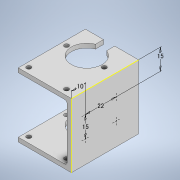
# Autodesk Inventor part: サーボモータ固定用２軸目3mm改_printer
Saved by Autodesk Inventor 2022 (Build 260153000, 153)
## iProperties
Created: 2022-11-23
Part Number: サーボモータ固定用２軸目3mm改_printer
Material: 一般
Document SubType Name: Modeling
Designer: tdn82
Density: 1 g/cm^3
Appearance: 既定
Author: tdn82
Autodesk Inventor part; units mm, degrees
ref_plane "YZ Plane" through (0, 0, 0) normal (1, 0, 0) x (0, 1, 0)
ref_plane "XZ Plane" through (0, 0, 0) normal (0, 1, 0) x (-1, 0, 0)
ref_plane "XY Plane" through (0, 0, 0) normal (0, 0, 1) x (1, 0, 0)
sketch "スケッチ1" plane through (0, 0, 0) normal (0, 1, 0) x (-1, 0, 0)
  line L0 (0, 0) -> (-38, 0)
  line L1 (-38, 0) -> (-38, -48)
  line L2 (-38, -48) -> (0, -48)
  line L3 (0, -48) -> (0, 0)
  dimension "d0" = 48
  dimension "d1" = 38
  constraints: 8 end point, 2 parallel, 1 horizontal, 1 perpendicular
  measures "d0" distance of L0.end L1.end
  measures "d1" distance of L1.end L2.end
extrude "押し出し1" add sketch "スケッチ1" along normal blind 46
sketch "スケッチ2" plane through (38, 0, -48) normal (0, 0, -1) x (-1, 0, 0)
  line L0 (3, 43) -> (59.072, 43)
  line L1 (59.072, 43) -> (59.072, 3)
  line L2 (59.072, 3) -> (3, 3)
  line L3 (3, 3) -> (3, 43)
  line L4 (0, 46) -> (38, 46) projected
  line L5 (0, 0) -> (38, 0) projected
  line L6 (0, 0) -> (0, 46) projected
  dimension "d4" = 40
  dimension "d6" = 3
  dimension "d7" = 3
  constraints: 8 end point, 2 parallel, 1 horizontal, 1 perpendicular
  measures "d4" distance of L2.end L0.start
  measures "d6" distance between parallel lines of L2 L5
  measures "d7" distance between parallel lines of L6 L3
extrude "押し出し2" cut sketch "スケッチ2" against normal blind 100
sketch "スケッチ3" plane through (0, 46, 0) normal (0, 1, 0) x (1, 0, 0)
  line L0 (38, 48) -> (0, 48) projected
  line L1 (38, 0) -> (38, 48) projected
  point P0 (0, 0)
  point P1 (17, 32)
  dimension "d10" = 16
  dimension "d11" = 21
  measures "d10" distance from line of L0 point (17, 32)
  measures "d11" distance from line of L1 point (17, 32)
hole "穴1" at (17, 46, -32) direction (0, -1, 0) diameter 22 end through all
sketch "スケッチ4" plane through (0, 46, 0) normal (0, 1, 0) x (1, 0, 0)
  line L0 (0, 0) -> (38, 0) projected
  line L1 (38, 0) -> (38, 48) projected
  point P0 (30.5, 4)
  point P1 (30.5, 31)
  point P2 (3.5, 4)
  point P3 (3.5, 31)
  point P4 (3.5, 4)
  dimension "d19" = 4
  dimension "d20" = 7.5
  dimension "d23" = 27
  dimension "d26" = 27
  constraints: 1 coincident, 1 horizontal, 1 vertical, 3 other
  measures "d19" distance from line of L0 point (30.5, 4)
  measures "d20" distance from line of L1 point (30.5, 4)
  measures "d23" distance of point (30.5, 4) point (30.5, 31)
  measures "d26" distance of point (30.5, 4) point (3.5, 4)
hole "穴2" at (30.5, 46, -4) at (30.5, 46, -31) at (3.5, 46, -31) at (3.5, 46, -4) direction (0, -1, 0) diameter 3.2 end through all
sketch "スケッチ6" plane through (38, 0, 0) normal (1, 0, 0) x (0, 0, -1)
  line L0 (0, 46) -> (48, 46) projected
  line L1 (0, 0) -> (0, 46) projected
  point P0 (10, 31)
  point P1 (32, 31)
  point P2 (10, 16)
  point P3 (32, 16)
  dimension "d45" = 15
  dimension "d46" = 10
  dimension "d49" = 22
  dimension "d52" = 15
  constraints: 1 horizontal, 1 vertical, 3 other
  measures "d45" distance from line of point (10, 31) L0
  measures "d46" distance from line of L1 point (10, 31)
  measures "d49" distance of point (10, 31) point (32, 31)
  measures "d52" distance of point (10, 31) point (10, 16)
fillet "フィレット1" radius 2 2 edges at (35, 3, -24) (35, 43, -24)
sketch "スケッチ7" plane through (0, 46, 0) normal (0, 1, 0) x (1, 0, 0)
  line L0 (38, 48) -> (0, 48) projected
  line L1 (13, 48) -> (21, 48)
  line L2 (21, 48) -> (21, 39.3329)
  line L3 (21, 39.3329) -> (13, 39.3329)
  line L4 (13, 39.3329) -> (13, 48)
  circle A0 centre (17, 32) radius 11 projected
  point P0 (0, 0)
  point P1 (13, 42.247)
  point P2 (21, 42.247)
  dimension "d69" = 8
  dimension "d70" = 4
  constraints: 8 end point, 2 parallel, 1 horizontal, 1 perpendicular, 1 point on line
  measures "d69" distance of L2.end L3.end
  measures "d70" distance from line of L4 A0.centre
extrude "押し出し3" cut sketch "スケッチ7" against normal blind 3 contours L2 A0 L4 L0
sketch "スケッチ8" plane through (35, 5, -48) normal (-1, 0, 0) x (0, 0, 1)
  line L0 (16, 11) -> (38, 11)
  line L1 (38, 11) -> (38, 26)
  line L2 (38, 26) -> (16, 26)
  line L3 (16, 26) -> (16, 11)
  line L4 (48, 36) -> (48, 0) projected
  line L5 (48, 41) -> (0, 41) projected
  point P0 (48, -5)
  dimension "d73" = 10
  dimension "d74" = 22
  dimension "d75" = 15
  dimension "d76" = 15
  constraints: 8 end point, 3 coincident, 2 parallel, 1 horizontal, 1 perpendicular
  measures "d73" distance between parallel lines of L4 L1
  measures "d74" distance of L0.start L0.end
  measures "d75" distance between parallel lines of L5 L2
  measures "d76" distance of L0.end L1.end
hole "穴5" at (35, 16, -10) at (35, 16, -32) at (35, 31, -32) at (35, 31, -10) direction (1, 0, 0) diameter 2.5 depth 0.1 tip angle 118
